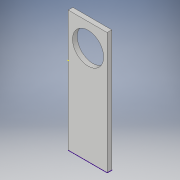
# Autodesk Inventor part: roller support
Saved by Autodesk Inventor 2019 (Build 230136000, 136)
## iProperties
Created: 2020-02-15
Part Number: roller support
Material: Generic
Document SubType Name: Modeling
Designer: Admin
Density: 1 g/cm^3
Appearance: Default
Author: Admin
Autodesk Inventor part; units mm, degrees
ref_plane "YZ Plane" through (0, 0, 0) normal (1, 0, 0) x (0, 1, 0)
ref_plane "XZ Plane" through (0, 0, 0) normal (0, 1, 0) x (-1, 0, 0)
ref_plane "XY Plane" through (0, 0, 0) normal (0, 0, 1) x (1, 0, 0)
sketch "Sketch1" plane through (0, 0, 0) normal (0, 0, 1) x (1, 0, 0)
  line L0 (0, 0) -> (0, 80)
  line L1 (0, 0) -> (25, 0)
  line L2 (25, 0) -> (25, 80)
  arc A0 (25, 80) -> (0, 80) centre (12.5, 58.3494) ccw
  dimension "d2" = 80
  dimension "d4" = 25
  dimension "d5" = 80
  dimension "d6" = 25
  constraints: 6 end point, 2 point on circle, 1 centre point, 1 horizontal, 1 perpendicular, 1 vertical
  measures "d2" distance of L0.start L0.end
  measures "d4" distance of L0.start L1.end
  measures "d5" distance of L1.end L2.end
  measures "d6" radius of A0
extrude "Extrusion1" add sketch "Sketch1" along normal blind 3
sketch "Sketch2" plane through (0, 0, 3) normal (0, 0, 1) x (1, 0, 0)
  circle A0 centre (12.5, 67.7859) radius 10
  point P0 (0, 0)
  dimension "d9" = 20
  constraints: 1 centre point
  measures "d9" diameter of A0
extrude "Extrusion2" cut sketch "Sketch2" against normal blind 3
sketch "Sketch3" plane through (0, 0, 0) normal (0, -1, 0) x (1, 0, 0)
  line L0 (25, 0) -> (0, 0) projected
  line L1 (25, 3) -> (0, 3) projected
  line L2 (0, 0) -> (25, 0)
  line L3 (25, 0) -> (25, 3)
  line L4 (25, 3) -> (0, 3)
  line L5 (0, 3) -> (0, 0)
  constraints: 8 end point, 2 parallel, 1 horizontal, 1 perpendicular
extrude "Extrusion3" add sketch "Sketch3" along normal blind 50
sketch "Sketch4" plane through (0, -50, 0) normal (0, -1, 0) x (1, 0, 0)
  line L0 (0, 0) -> (0, 3) projected
  line L1 (25, 0) -> (25, 3) projected
  line L2 (0, 3) -> (25, 3)
  line L3 (25, 3) -> (25, 0)
  line L4 (25, 0) -> (0, 0)
  line L5 (0, 0) -> (0, 3)
  constraints: 8 end point, 2 parallel, 1 horizontal, 1 perpendicular
sketch "Sketch5" plane through (0, 0, 3) normal (0, 0, 1) x (1, 0, 0)
  circle A0 centre (12.7766, 13.1416) radius 10
  point P0 (0, 0)
  dimension "d14" = 20
  constraints: 1 centre point
  measures "d14" diameter of A0
extrude "Extrusion4" cut sketch "Sketch5" against normal blind 50
sketch "Sketch6" plane through (0, 0, 3) normal (0, 0, 1) x (1, 0, 0)
  line L0 (31.6061, 27.9408) -> (-29.0129, 27.9408)
  line L1 (-29.0129, 27.9408) -> (-29.0129, 90.0456)
  line L2 (-29.0129, 90.0456) -> (31.6061, 90.0456)
  line L3 (31.6061, 90.0456) -> (31.6061, 27.9408)
  point P0 (0, 0)
  constraints: 8 end point, 2 parallel, 1 horizontal, 1 perpendicular
extrude "Extrusion5" cut sketch "Sketch6" against normal blind 50
sketch "Sketch7" plane through (0, 0, 3) normal (0, 0, 1) x (1, 0, 0)
  point P0 (0, 0)
body "Solid1"
